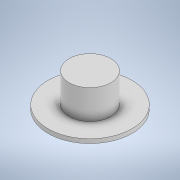
# Autodesk Inventor part: just_ring
Saved by Autodesk Inventor 2021 (Build 250183000, 183)
## iProperties
Created: 2021-03-25
Part Number: just_ring
Material: Generic
Document SubType Name: Modeling
Designer: Patrick
Density: 1 g/cm^3
Appearance: Default
Author: Patrick
Autodesk Inventor part; units mm, degrees
ref_plane "YZ Plane" through (0, 0, 0) normal (1, 0, 0) x (0, 1, 0)
ref_plane "XZ Plane" through (0, 0, 0) normal (0, 1, 0) x (-1, 0, 0)
ref_plane "XY Plane" through (0, 0, 0) normal (0, 0, 1) x (1, 0, 0)
sketch "Sketch1" plane through (0, 0, 0) normal (0, 1, 0) x (-1, 0, 0)
  line L0 (-12.3843, -4.2113) -> (-12.8886, -4.5987)
  line L1 (-12.8886, -4.5987) -> (-13.9876, -5.4968)
  line L2 (-13.9876, -5.4968) -> (-14.4681, -5.9314)
  line L3 (-14.4681, -5.9314) -> (-15.4677, -6.9308)
  line L4 (-15.4677, -6.9308) -> (-15.9089, -7.3994)
  line L5 (-15.9089, -7.3994) -> (-16.7645, -8.4419)
  line L6 (-16.7645, -8.4419) -> (-17.1543, -8.9265)
  line L7 (-17.1543, -8.9265) -> (-17.5075, -9.4417)
  line L8 (-17.5075, -9.4417) -> (-18.2559, -10.5566)
  line L9 (-18.2559, -10.5566) -> (-18.5835, -11.1249)
  line L10 (-18.5835, -11.1249) -> (-19.2428, -12.3521)
  line L11 (-19.2428, -12.3521) -> (-19.53, -12.9576)
  line L12 (-19.53, -12.9576) -> (-20.0599, -14.2366)
  line L13 (-20.0599, -14.2366) -> (-20.2967, -14.8606)
  line L14 (-20.2967, -14.8606) -> (-20.6795, -16.1223)
  line L15 (-20.6795, -16.1223) -> (-20.8609, -16.7425)
  line L16 (-20.8609, -16.7425) -> (-20.9954, -17.3785)
  line L17 (-20.9954, -17.3785) -> (-21.2538, -18.6633)
  line L18 (-21.2538, -18.6633) -> (-21.3426, -19.3412)
  line L19 (-21.3426, -19.3412) -> (-21.4785, -20.692)
  line L20 (-21.4785, -20.692) -> (-21.5136, -21.3905)
  line L21 (-21.5136, -21.3905) -> (-21.5137, -22.738)
  line L22 (-21.5137, -22.738) -> (-21.4928, -23.4347)
  line L23 (-21.4928, -23.4347) -> (-21.3671, -24.7106)
  line L24 (-21.3671, -24.7106) -> (-21.2943, -25.3819)
  line L25 (-21.2943, -25.3819) -> (-21.1697, -26.05)
  line L26 (-21.1697, -26.05) -> (-20.924, -27.2994)
  line L27 (-20.924, -27.2994) -> (-20.7385, -27.9897)
  line L28 (-20.7385, -27.9897) -> (-20.3585, -29.2522)
  line L29 (-20.3585, -29.2522) -> (-20.113, -29.9406)
  line L30 (-20.113, -29.9406) -> (-19.6123, -31.1495)
  line L31 (-19.6123, -31.1495) -> (-19.3137, -31.8134)
  line L32 (-19.3137, -31.8134) -> (-18.7268, -32.9115)
  line L33 (-18.7268, -32.9115) -> (-18.3886, -33.5296)
  line L34 (-18.3886, -33.5296) -> (-18.0019, -34.1235)
  line L35 (-18.0019, -34.1235) -> (-17.3169, -35.1534)
  line L36 (-17.3169, -35.1534) -> (-16.8634, -35.7437)
  line L37 (-16.8634, -35.7437) -> (-16.0525, -36.7361)
  line L38 (-16.0525, -36.7361) -> (-15.5427, -37.2997)
  line L39 (-15.5427, -37.2997) -> (-14.6425, -38.2)
  line L40 (-14.6425, -38.2) -> (-14.0924, -38.718)
  line L41 (-14.0924, -38.718) -> (-13.1548, -39.4876)
  line L42 (-13.1548, -39.4876) -> (-12.5861, -39.945)
  line L43 (-12.5861, -39.945) -> (-11.9815, -40.3595)
  line L44 (-11.9815, -40.3595) -> (-10.9796, -41.032)
  line L45 (-10.9796, -41.032) -> (-10.3141, -41.4157)
  line L46 (-10.3141, -41.4157) -> (-9.2107, -42.0085)
  line L47 (-9.2107, -42.0085) -> (-8.5039, -42.3437)
  line L48 (-8.5039, -42.3437) -> (-7.352, -42.8209)
  line L49 (-7.352, -42.8209) -> (-6.6268, -43.0961)
  line L50 (-6.6268, -43.0961) -> (-5.4874, -43.4417)
  line L51 (-5.4874, -43.4417) -> (-4.7703, -43.6516)
  line L52 (-4.7703, -43.6516) -> (-4.0375, -43.8064)
  line L53 (-4.0375, -43.8064) -> (-2.8737, -44.0405)
  line L54 (-2.8737, -44.0405) -> (-2.0978, -44.1421)
  line L55 (-2.0978, -44.1421) -> (-0.8683, -44.2658)
  line L56 (-0.8683, -44.2658) -> (-0.0749, -44.3057)
  line L57 (-0.0749, -44.3057) -> (1.1588, -44.3057)
  line L58 (1.1588, -44.3057) -> (1.9436, -44.2821)
  line L59 (1.9436, -44.2821) -> (3.1195, -44.1663)
  line L60 (3.1195, -44.1663) -> (3.869, -44.0851)
  line L61 (3.869, -44.0851) -> (4.6101, -43.9468)
  line L62 (4.6101, -43.9468) -> (5.7695, -43.7187)
  line L63 (5.7695, -43.7187) -> (6.5277, -43.5151)
  line L64 (6.5277, -43.5151) -> (7.709, -43.1594)
  line L65 (7.709, -43.1594) -> (8.4572, -42.8926)
  line L66 (8.4572, -42.8926) -> (9.5989, -42.4197)
  line L67 (9.5989, -42.4197) -> (10.3125, -42.0987)
  line L68 (10.3125, -42.0987) -> (11.3595, -41.539)
  line L69 (11.3595, -41.539) -> (12.0166, -41.1795)
  line L70 (12.0166, -41.1795) -> (12.6427, -40.7719)
  line L71 (12.6427, -40.7719) -> (13.6341, -40.1124)
  line L72 (13.6341, -40.1124) -> (14.2492, -39.6398)
  line L73 (14.2492, -39.6398) -> (15.2146, -38.8508)
  line L74 (15.2146, -38.8508) -> (15.7948, -38.3261)
  line L75 (15.7948, -38.3261) -> (16.6804, -37.4404)
  line L76 (16.6804, -37.4404) -> (17.2071, -36.8811)
  line L77 (17.2071, -36.8811) -> (17.9726, -35.9484)
  line L78 (17.9726, -35.9484) -> (18.4321, -35.3772)
  line L79 (18.4321, -35.3772) -> (18.8448, -34.7753)
  line L80 (18.8448, -34.7753) -> (19.5207, -33.7681)
  line L81 (19.5207, -33.7681) -> (19.8981, -33.1135)
  line L82 (19.8981, -33.1135) -> (20.5006, -31.992)
  line L83 (20.5006, -31.992) -> (20.8262, -31.3053)
  line L84 (20.8262, -31.3053) -> (21.3166, -30.1212)
  line L85 (21.3166, -30.1212) -> (21.5808, -29.4252)
  line L86 (21.5808, -29.4252) -> (21.9398, -28.2416)
  line L87 (21.9398, -28.2416) -> (22.1389, -27.5614)
  line L88 (22.1389, -27.5614) -> (22.2845, -26.8721)
  line L89 (22.2845, -26.8721) -> (22.53, -25.6515)
  line L90 (22.53, -25.6515) -> (22.6245, -24.9296)
  line L91 (22.6245, -24.9296) -> (22.7554, -23.6277)
  line L92 (22.7554, -23.6277) -> (22.7921, -22.8978)
  line L93 (22.7921, -22.8978) -> (22.792, -21.5793)
  line L94 (22.792, -21.5793) -> (22.7706, -20.8649)
  line L95 (22.7706, -20.8649) -> (22.6458, -19.5976)
  line L96 (22.6458, -19.5976) -> (22.5725, -18.922)
  line L97 (22.5725, -18.922) -> (22.4487, -18.2583)
  line L98 (22.4487, -18.2583) -> (22.2012, -17.0003)
  line L99 (22.2012, -17.0003) -> (22.0204, -16.3271)
  line L100 (22.0204, -16.3271) -> (21.6318, -15.0368)
  line L101 (21.6318, -15.0368) -> (21.3969, -14.3781)
  line L102 (21.3969, -14.3781) -> (20.8773, -13.1238)
  line L103 (20.8773, -13.1238) -> (20.5968, -12.5003)
  line L104 (20.5968, -12.5003) -> (19.979, -11.3445)
  line L105 (19.979, -11.3445) -> (19.667, -10.7743)
  line L106 (19.667, -10.7743) -> (19.3144, -10.2327)
  line L107 (19.3144, -10.2327) -> (18.5842, -9.135)
  line L108 (18.5842, -9.135) -> (18.1776, -8.6057)
  line L109 (18.1776, -8.6057) -> (17.3015, -7.5337)
  line L110 (17.3015, -7.5337) -> (16.852, -7.0367)
  line L111 (16.852, -7.0367) -> (15.8669, -6.0517)
  line L112 (15.8669, -6.0517) -> (15.3893, -5.6019)
  line L113 (15.3893, -5.6019) -> (14.3514, -4.7501)
  line L114 (14.3514, -4.7501) -> (13.8646, -4.3586)
  line L115 (13.8646, -4.3586) -> (13.3517, -4.0069)
  line L116 (13.3517, -4.0069) -> (12.2319, -3.2553)
  line L117 (12.2319, -3.2553) -> (11.6743, -2.9339)
  line L118 (11.6743, -2.9339) -> (10.429, -2.265)
  line L119 (10.429, -2.265) -> (9.8436, -1.9874)
  line L120 (9.8436, -1.9874) -> (8.5324, -1.4443)
  line L121 (8.5324, -1.4443) -> (7.9378, -1.2186)
  line L122 (7.9378, -1.2186) -> (6.6316, -0.8224)
  line L123 (6.6316, -0.8224) -> (6.0605, -0.6553)
  arc A0 (6.0605, -0.6553) -> (6.0364, -0.6492) centre (0.6401, -22.1587) ccw
  line L124 (6.0364, -0.6492) -> (5.4558, -0.5265)
  line L125 (5.4558, -0.5265) -> (4.1145, -0.2568)
  line L126 (4.1145, -0.2568) -> (3.4905, -0.175)
  line L127 (3.4905, -0.175) -> (2.0674, -0.0319)
  line L128 (2.0674, -0.0319) -> (1.4324, 0)
  line L129 (1.4324, 0) -> (0, 0)
  line L130 (0, 0) -> (-0.6263, -0.0188)
  line L131 (-0.6263, -0.0188) -> (-1.9935, -0.1534)
  line L132 (-1.9935, -0.1534) -> (-2.5641, -0.2153)
  arc A1 (-2.5641, -0.2153) -> (-2.6174, -0.2232) centre (0.6401, -22.1587) ccw
  line L133 (-2.6174, -0.2232) -> (-3.1816, -0.3284)
  line L134 (-3.1816, -0.3284) -> (-4.5296, -0.5936)
  line L135 (-4.5296, -0.5936) -> (-5.1348, -0.7562)
  line L136 (-5.1348, -0.7562) -> (-6.5063, -1.1691)
  line L137 (-6.5063, -1.1691) -> (-7.1052, -1.3826)
  line L138 (-7.1052, -1.3826) -> (-8.4267, -1.93)
  line L139 (-8.4267, -1.93) -> (-9.0006, -2.1881)
  line L140 (-9.0006, -2.1881) -> (-10.2071, -2.833)
  line L141 (-10.2071, -2.833) -> (-10.7278, -3.1179)
  arc A2 (-10.7278, -3.1179) -> (-10.7491, -3.1307) centre (0.6401, -22.1587) ccw
  line L142 (-10.7491, -3.1307) -> (-11.2478, -3.4553)
  line L143 (-11.2478, -3.4553) -> (-12.3843, -4.2113)
  circle A3 centre (0.6401, -22.1587) radius 12.65
  circle A4 centre (-8.5804, -37.3303) radius 4.2966
  circle A5 centre (-14.9309, -30.6874) radius 4.2966
  circle A6 centre (-17.1092, -21.7593) radius 4.2966
  circle A7 centre (-14.5315, -12.9382) radius 4.2966
  circle A8 centre (0.2407, -39.9079) radius 4.2966
  circle A9 centre (9.1688, -37.7296) radius 4.2966
  circle A10 centre (15.8117, -31.3791) radius 4.2966
  circle A11 centre (1.0394, -4.4094) radius 4.2966
  circle A12 centre (-7.8887, -6.5877) radius 4.2966
  circle A13 centre (9.8605, -6.9871) radius 4.2966
  circle A14 centre (18.3893, -22.558) radius 4.2966
  circle A15 centre (16.211, -13.6299) radius 4.2966
  point P0 (0, 0)
  point P1 (0.6401, -22.1587)
  dimension "d12" = 25.3
  constraints: 288 end point, 16 centre point, 6 point on circle
  measures "d12" diameter of A3
extrude "Extrusion4" add sketch "Sketch1" along normal blind 17.78 contours A3
sketch "Sketch5" plane through (-0.6401, 0, -22.1587) normal (0, -1, 0) x (1, 0, 0)
  circle A0 centre (0, 0) radius 25.4
  point P0 (0.6401, 22.1587)
  dimension "d15" = 50.8
  constraints: 1 centre point
  measures "d15" diameter of A0
extrude "Extrusion5" add sketch "Sketch5" along normal blind 2.54
body "Solid2"
